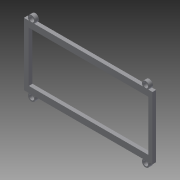
# Autodesk Inventor part: lcd-spacer-model
Saved by Autodesk Inventor 2014 (Build 180170000, 170)
## iProperties
Created: 2014-07-20
Part Number: lcd-spacer-model
Material: Generic
Document SubType Name: Modeling
Designer: james
Density: 1 g/cm^3
Appearance: Default
Author: james
Autodesk Inventor part; units mm, degrees
ref_plane "YZ Plane" through (0, 0, 0) normal (1, 0, 0) x (0, 1, 0)
ref_plane "XZ Plane" through (0, 0, 0) normal (0, 1, 0) x (-1, 0, 0)
ref_plane "XY Plane" through (0, 0, 0) normal (0, 0, 1) x (1, 0, 0)
sketch "Sketch1" plane through (0, 0, 0) normal (0, 1, 0) x (-1, 0, 0)
  spline S0 degree 3 poles (-9.8463, -11.5333) (-9.7942, -11.6131) (-9.7348, -11.6874) (-9.6692, -11.7553) (-9.4724, -11.9589) (-9.2192, -12.1042) (-8.936, -12.1641) (-8.8416, -12.1841) (-8.7439, -12.1946) (-8.6437, -12.1946) (-8.5436, -12.1946) (-8.4459, -12.1841) (-8.3515, -12.1641) (-8.0682, -12.1042) (-7.8151, -11.9589) (-7.6183, -11.7553) (-7.5527, -11.6874) (-7.4933, -11.6131) (-7.4412, -11.5333) (-7.337, -11.3737) (-7.2616, -11.1922) (-7.223, -10.9969) (-7.2037, -10.8993) (-7.1935, -10.7982) (-7.1935, -10.6946) (-7.1935, -9.8662) (-7.8428, -9.1946) (-8.6437, -9.1946) (-9.4447, -9.1946) (-10.094, -9.8662) (-10.094, -10.6946) (-10.094, -10.7982) (-10.0838, -10.8993) (-10.0645, -10.9969) (-10.0259, -11.1922) (-9.9505, -11.3737) (-9.8463, -11.5333) knots 0 0 0 0 1 1 1 2 2 2 3 3 3 4 4 4 5 5 5 6 6 6 7 7 7 8 8 8 9 9 9 10 10 10 11 11 11 12 12 12 12
  line L0 (-9.8463, -11.5333) -> (-9.7942, -11.6131) construction
  line L1 (-9.7942, -11.6131) -> (-9.7348, -11.6874) construction
  line L2 (-9.7348, -11.6874) -> (-9.6692, -11.7553) construction
  line L3 (-9.6692, -11.7553) -> (-9.4724, -11.9589) construction
  line L4 (-9.4724, -11.9589) -> (-9.2192, -12.1042) construction
  line L5 (-9.2192, -12.1042) -> (-8.936, -12.1641) construction
  line L6 (-8.936, -12.1641) -> (-8.8416, -12.1841) construction
  line L7 (-8.8416, -12.1841) -> (-8.7439, -12.1946) construction
  line L8 (-8.7439, -12.1946) -> (-8.6437, -12.1946) construction
  line L9 (-8.6437, -12.1946) -> (-8.5436, -12.1946) construction
  line L10 (-8.5436, -12.1946) -> (-8.4459, -12.1841) construction
  line L11 (-8.4459, -12.1841) -> (-8.3515, -12.1641) construction
  line L12 (-8.3515, -12.1641) -> (-8.0682, -12.1042) construction
  line L13 (-8.0682, -12.1042) -> (-7.8151, -11.9589) construction
  line L14 (-7.8151, -11.9589) -> (-7.6183, -11.7553) construction
  line L15 (-7.6183, -11.7553) -> (-7.5527, -11.6874) construction
  line L16 (-7.5527, -11.6874) -> (-7.4933, -11.6131) construction
  line L17 (-7.4933, -11.6131) -> (-7.4412, -11.5333) construction
  line L18 (-7.4412, -11.5333) -> (-7.337, -11.3737) construction
  line L19 (-7.337, -11.3737) -> (-7.2616, -11.1922) construction
  line L20 (-7.2616, -11.1922) -> (-7.223, -10.9969) construction
  line L21 (-7.223, -10.9969) -> (-7.2037, -10.8993) construction
  line L22 (-7.2037, -10.8993) -> (-7.1935, -10.7982) construction
  line L23 (-7.1935, -10.7982) -> (-7.1935, -10.6946) construction
  line L24 (-7.1935, -10.6946) -> (-7.1935, -9.8662) construction
  line L25 (-7.1935, -9.8662) -> (-7.8428, -9.1946) construction
  line L26 (-7.8428, -9.1946) -> (-8.6437, -9.1946) construction
  line L27 (-8.6437, -9.1946) -> (-9.4447, -9.1946) construction
  line L28 (-9.4447, -9.1946) -> (-10.094, -9.8662) construction
  line L29 (-10.094, -9.8662) -> (-10.094, -10.6946) construction
  line L30 (-10.094, -10.6946) -> (-10.094, -10.7982) construction
  line L31 (-10.094, -10.7982) -> (-10.0838, -10.8993) construction
  line L32 (-10.0838, -10.8993) -> (-10.0645, -10.9969) construction
  line L33 (-10.0645, -10.9969) -> (-10.0259, -11.1922) construction
  line L34 (-10.0259, -11.1922) -> (-9.9505, -11.3737) construction
  line L35 (-9.9505, -11.3737) -> (-9.8463, -11.5333) construction
  spline S1 degree 3 poles (83.1689, -11.5333) (83.221, -11.6131) (83.2803, -11.6874) (83.3459, -11.7553) (83.5428, -11.9589) (83.7959, -12.1042) (84.0791, -12.1641) (84.1735, -12.1841) (84.2713, -12.1946) (84.3714, -12.1946) (84.4715, -12.1946) (84.5693, -12.1841) (84.6637, -12.1641) (84.9469, -12.1042) (85.2001, -11.9589) (85.3969, -11.7553) (85.4625, -11.6874) (85.5218, -11.6131) (85.574, -11.5333) (85.6782, -11.3737) (85.7536, -11.1922) (85.7922, -10.9969) (85.8115, -10.8993) (85.8217, -10.7982) (85.8217, -10.6946) (85.8217, -9.8662) (85.1724, -9.1946) (84.3714, -9.1946) (83.5705, -9.1946) (82.9212, -9.8662) (82.9212, -10.6946) (82.9212, -10.7982) (82.9313, -10.8993) (82.9506, -10.9969) (82.9893, -11.1922) (83.0646, -11.3737) (83.1689, -11.5333) knots 0 0 0 0 1 1 1 2 2 2 3 3 3 4 4 4 5 5 5 6 6 6 7 7 7 8 8 8 9 9 9 10 10 10 11 11 11 12 12 12 12
  line L36 (83.1689, -11.5333) -> (83.221, -11.6131) construction
  line L37 (83.221, -11.6131) -> (83.2803, -11.6874) construction
  line L38 (83.2803, -11.6874) -> (83.3459, -11.7553) construction
  line L39 (83.3459, -11.7553) -> (83.5428, -11.9589) construction
  line L40 (83.5428, -11.9589) -> (83.7959, -12.1042) construction
  line L41 (83.7959, -12.1042) -> (84.0791, -12.1641) construction
  line L42 (84.0791, -12.1641) -> (84.1735, -12.1841) construction
  line L43 (84.1735, -12.1841) -> (84.2713, -12.1946) construction
  line L44 (84.2713, -12.1946) -> (84.3714, -12.1946) construction
  line L45 (84.3714, -12.1946) -> (84.4715, -12.1946) construction
  line L46 (84.4715, -12.1946) -> (84.5693, -12.1841) construction
  line L47 (84.5693, -12.1841) -> (84.6637, -12.1641) construction
  line L48 (84.6637, -12.1641) -> (84.9469, -12.1042) construction
  line L49 (84.9469, -12.1042) -> (85.2001, -11.9589) construction
  line L50 (85.2001, -11.9589) -> (85.3969, -11.7553) construction
  line L51 (85.3969, -11.7553) -> (85.4625, -11.6874) construction
  line L52 (85.4625, -11.6874) -> (85.5218, -11.6131) construction
  line L53 (85.5218, -11.6131) -> (85.574, -11.5333) construction
  line L54 (85.574, -11.5333) -> (85.6782, -11.3737) construction
  line L55 (85.6782, -11.3737) -> (85.7536, -11.1922) construction
  line L56 (85.7536, -11.1922) -> (85.7922, -10.9969) construction
  line L57 (85.7922, -10.9969) -> (85.8115, -10.8993) construction
  line L58 (85.8115, -10.8993) -> (85.8217, -10.7982) construction
  line L59 (85.8217, -10.7982) -> (85.8217, -10.6946) construction
  line L60 (85.8217, -10.6946) -> (85.8217, -9.8662) construction
  line L61 (85.8217, -9.8662) -> (85.1724, -9.1946) construction
  line L62 (85.1724, -9.1946) -> (84.3714, -9.1946) construction
  line L63 (84.3714, -9.1946) -> (83.5705, -9.1946) construction
  line L64 (83.5705, -9.1946) -> (82.9212, -9.8662) construction
  line L65 (82.9212, -9.8662) -> (82.9212, -10.6946) construction
  line L66 (82.9212, -10.6946) -> (82.9212, -10.7982) construction
  line L67 (82.9212, -10.7982) -> (82.9313, -10.8993) construction
  line L68 (82.9313, -10.8993) -> (82.9506, -10.9969) construction
  line L69 (82.9506, -10.9969) -> (82.9893, -11.1922) construction
  line L70 (82.9893, -11.1922) -> (83.0646, -11.3737) construction
  line L71 (83.0646, -11.3737) -> (83.1689, -11.5333) construction
  line L72 (-14.2577, -12.5451) -> (-14.2577, -64.0273)
  line L73 (-14.2577, -64.0273) -> (90.783, -64.0273)
  line L74 (90.783, -64.0273) -> (90.783, -12.5451)
  line L75 (90.783, -12.5451) -> (-14.2577, -12.5451)
  spline S2 degree 3 poles (-8.6437, -64.2555) (-9.4447, -64.2555) (-10.094, -64.9271) (-10.094, -65.7555) (-10.094, -66.5839) (-9.4447, -67.2555) (-8.6437, -67.2555) (-7.8428, -67.2555) (-7.1935, -66.5839) (-7.1935, -65.7555) (-7.1935, -64.9271) (-7.8428, -64.2555) (-8.6437, -64.2555) knots 0 0 0 0 1 1 1 2 2 2 3 3 3 4 4 4 4
  line L76 (-8.6437, -64.2555) -> (-9.4447, -64.2555) construction
  line L77 (-9.4447, -64.2555) -> (-10.094, -64.9271) construction
  line L78 (-10.094, -64.9271) -> (-10.094, -65.7555) construction
  line L79 (-10.094, -65.7555) -> (-10.094, -66.5839) construction
  line L80 (-10.094, -66.5839) -> (-9.4447, -67.2555) construction
  line L81 (-9.4447, -67.2555) -> (-8.6437, -67.2555) construction
  line L82 (-8.6437, -67.2555) -> (-7.8428, -67.2555) construction
  line L83 (-7.8428, -67.2555) -> (-7.1935, -66.5839) construction
  line L84 (-7.1935, -66.5839) -> (-7.1935, -65.7555) construction
  line L85 (-7.1935, -65.7555) -> (-7.1935, -64.9271) construction
  line L86 (-7.1935, -64.9271) -> (-7.8428, -64.2555) construction
  line L87 (-7.8428, -64.2555) -> (-8.6437, -64.2555) construction
  spline S3 degree 3 poles (84.4193, -64.2555) (83.6184, -64.2555) (82.9691, -64.9271) (82.9691, -65.7555) (82.9691, -66.5839) (83.6184, -67.2555) (84.4193, -67.2555) (85.2203, -67.2555) (85.8695, -66.5839) (85.8695, -65.7555) (85.8695, -64.9271) (85.2203, -64.2555) (84.4193, -64.2555) knots 0 0 0 0 1 1 1 2 2 2 3 3 3 4 4 4 4
  line L88 (84.4193, -64.2555) -> (83.6184, -64.2555) construction
  line L89 (83.6184, -64.2555) -> (82.9691, -64.9271) construction
  line L90 (82.9691, -64.9271) -> (82.9691, -65.7555) construction
  line L91 (82.9691, -65.7555) -> (82.9691, -66.5839) construction
  line L92 (82.9691, -66.5839) -> (83.6184, -67.2555) construction
  line L93 (83.6184, -67.2555) -> (84.4193, -67.2555) construction
  line L94 (84.4193, -67.2555) -> (85.2203, -67.2555) construction
  line L95 (85.2203, -67.2555) -> (85.8695, -66.5839) construction
  line L96 (85.8695, -66.5839) -> (85.8695, -65.7555) construction
  line L97 (85.8695, -65.7555) -> (85.8695, -64.9271) construction
  line L98 (85.8695, -64.9271) -> (85.2203, -64.2555) construction
  line L99 (85.2203, -64.2555) -> (84.4193, -64.2555) construction
  point P0 (0, 0)
  constraints: 8 end point, 8 other
sketch "Sketch2" plane through (0, 0, 0) normal (0, 1, 0) x (-1, 0, 0)
  circle A0 centre (84.4532, -10.6585) radius 2
  circle A1 centre (-8.5926, -10.6585) radius 2
  circle A2 centre (-8.5926, -65.7836) radius 2
  circle A3 centre (84.4532, -65.7836) radius 2
  circle A4 centre (-8.5926, -10.6585) radius 3
  circle A5 centre (-8.5926, -65.7836) radius 3
  circle A6 centre (84.4532, -65.7836) radius 3
  circle A7 centre (84.4532, -10.6585) radius 3
  line L0 (-14.1634, -12.6585) -> (90.7016, -12.6585)
  line L1 (90.7016, -12.6585) -> (90.7016, -17.6585)
  line L2 (90.7016, -17.6585) -> (-14.1634, -17.6585)
  line L3 (-14.1634, -17.6585) -> (-14.1634, -12.6585)
  line L4 (90.7016, -63.7836) -> (-14.1634, -63.7836)
  line L5 (-14.1634, -63.7836) -> (-14.1634, -58.7836)
  line L6 (-14.1634, -58.7836) -> (90.7016, -58.7836)
  line L7 (90.7016, -58.7836) -> (90.7016, -63.7836)
  line L8 (-14.1634, -12.6585) -> (-10.8287, -12.6585)
  line L9 (-10.8287, -12.6585) -> (-10.8287, -63.7836)
  line L10 (-10.8287, -63.7836) -> (-14.1634, -63.7836)
  line L11 (-14.1634, -63.7836) -> (-14.1634, -12.6585)
  line L12 (86.6893, -12.6585) -> (90.7016, -12.6585)
  line L13 (90.7016, -12.6585) -> (90.7016, -63.7836)
  line L14 (90.7016, -63.7836) -> (86.6893, -63.7836)
  line L15 (86.6893, -63.7836) -> (86.6893, -12.6585)
  point P0 (0, 0)
  dimension "d5" = 6
  dimension "d7" = 6
  dimension "d0" = 4
  dimension "d1" = 4
  dimension "d2" = 4
  dimension "d3" = 4
  dimension "d4" = 6
  dimension "d6" = 6
  dimension "d8" = 5
  dimension "d9" = 5
  constraints: 32 end point, 8 parallel, 6 centre point, 4 coincident, 4 horizontal, 4 perpendicular, 2 point on line, 6 other
  measures "d0" diameter of A0
  measures "d1" diameter of A1
  measures "d2" diameter of A2
  measures "d3" diameter of A3
  measures "d4" diameter of A4
  measures "d6" diameter of A6
  measures "d8" distance of L0.end L1.end
  measures "d9" distance of L4.end L5.end
extrude "Extrusion1" add sketch "Sketch2" along normal blind 3 contours L0 A7 | L0 A7 | A7 L15 L2 L9 A4 L0 | L0 L1 L2 L15 | L0 A4 | A4 L0 | L2 L13 L6 L15 | L9 L2 L3 L0 | L9 L6 L11 L2 | L15 A6 L4 A5 L9 L6 | L6 L7 L4 L15 | L9 L4 L5 L6 | L4 A6 | A6 L4 | L4 A5 | A5 L4
body "Solid1"
